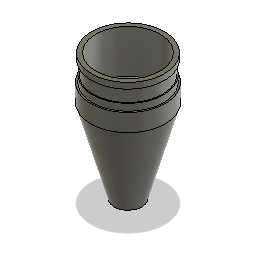
Lazer_Engraver_Nozzle (Autodesk Fusion 360 design; units mm, degrees)
Autodesk Fusion 360 part; units mm, degrees
sketch "Sketch1" plane through (0, 0, 0) normal (0, 0, 1) x (1, 0, 0)
  line L0 (0, 0) -> (-9.144, 0)
  line L1 (-9.144, 0) -> (-9.144, -1.4732)
  line L2 (-9.144, -1.4732) -> (-8.6614, -1.4732)
  line L3 (-8.6614, -1.4732) -> (-8.6614, -4.7244)
  line L4 (-8.6614, -4.7244) -> (-8.9154, -4.7244)
  line L5 (-8.9154, -4.7244) -> (-8.9154, -6.4262)
  line L6 (-8.9154, -6.4262) -> (-9.3218, -6.4262)
  line L7 (-9.3218, -6.4262) -> (-9.3218, -10.8189)
  line L8 (0, 0) -> (0, -32.766)
  line L9 (-1.7145, -32.766) -> (-3.4925, -31.7892)
  line L10 (-9.3218, -10.8189) -> (-3.4925, -31.7892)
  line L11 (-9.3218, -9.6713) -> (-8.0518, -9.6713)
  line L12 (-7.8884, -15.9752) -> (-6.6648, -15.6351)
  line L13 (-8.0518, 0) -> (-8.0518, -10.8189)
  line L14 (-3.4925, -31.7892) -> (-2.2689, -31.449)
  line L15 (-2.2689, -31.449) -> (-6.6648, -15.6351)
  line L16 (-8.0518, -9.6713) -> (-8.0518, -10.8189)
  line L17 (-6.6648, -15.6351) -> (-8.0518, -10.8189)
  line L18 (-2.2689, -31.449) -> (-1.7145, -32.766)
  dimension "d15" = 0.4064
  dimension "d16" = 1.7145
  dimension "d17" = 1.778
  dimension "d18" = 20.9703
  dimension "d19" = 1.27
  dimension "d20" = 1.27
  dimension "d22" = 1.27
  constraint coincident L0.start L8.start
  constraint horizontal L0
  constraint perpendicular L0 L1
  constraint perpendicular L1 L2
  constraint perpendicular L2 L3
  constraint horizontal L4
  constraint perpendicular L4 L5
  constraint horizontal L6
  constraint perpendicular L6 L7
  constraint perpendicular L0 L8
  constraint coincident L7 L11.start
  constraint perpendicular L7 L11
  constraint coincident L10 L12.start
  constraint perpendicular L10 L12
  constraint coincident L0 L13.start
  constraint perpendicular L11 L13
  constraint perpendicular L10 L14
  constraint perpendicular L11 L16
  measures "d15" distance of L5.end L6.end
  measures "d16" distance of L8.end L9.start
  measures "d17" horizontal distance of L9.end L9.start
  measures "d18" vertical distance of L7.end L9.end
  measures "d19" distance of L11.start L11.end
  measures "d20" distance of L12.start L12.end
  measures "d22" distance of L9.end L14.end
revolve "Revolve1" add sketch "Sketch1" angle 360 about axis through (0, 0, 0) along (0, -1, 0)
equation "d16 = ( 0.135 / 2 ) * 1 in"
